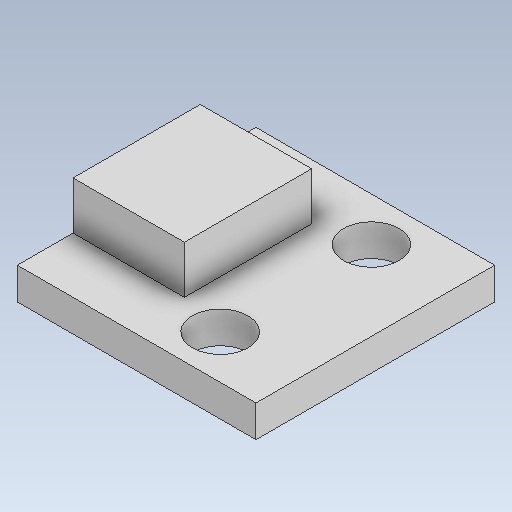
# Autodesk Inventor part: Charger_Port
Saved by Autodesk Inventor 2020 (Build 240168000, 168)
## iProperties
Created: 2021-11-16
Part Number: Charger_Port
Material: Generic
Document SubType Name: Modeling
Designer: mtkts
Density: 1 g/cm^3
Appearance: Default
Author: mtkts
Autodesk Inventor part; units mm, degrees
ref_plane "YZ Plane" through (0, 0, 0) normal (1, 0, 0) x (0, 1, 0)
ref_plane "XZ Plane" through (0, 0, 0) normal (0, 1, 0) x (-1, 0, 0)
ref_plane "XY Plane" through (0, 0, 0) normal (0, 0, 1) x (1, 0, 0)
sketch "Sketch1" plane through (0, 0, 0) normal (0, 1, 0) x (-1, 0, 0)
  line L0 (-7.5, 7.5) -> (7.5, 7.5)
  line L1 (7.5, 7.5) -> (7.5, -7.5)
  line L2 (7.5, -7.5) -> (-7.5, -7.5)
  line L3 (-7.5, -7.5) -> (-7.5, 7.5)
  line L4 (-7.5, 7.5) -> (7.5, -7.5) construction
  line L5 (7.5, 7.5) -> (-7.5, -7.5) construction
  point P0 (0, 0)
  dimension "d0" = 15
  dimension "d1" = 15
  constraints: 12 end point, 2 midpoint, 2 parallel, 1 horizontal, 1 perpendicular
  measures "d0" distance of L1.end L2.end
  measures "d1" distance of L0.end L1.end
extrude "Extrusion1" add sketch "Sketch1" along normal blind 2
sketch "Sketch2" plane through (0, 2, 0) normal (0, 1, 0) x (1, 0, 0)
  line L0 (7.5, 7.5) -> (-7.5, 7.5) construction
  line L1 (-7.5, 7.5) -> (-7.5, -7.5) construction
  line L2 (-7.5, -7.5) -> (7.5, -7.5) construction
  line L3 (7.5, -7.5) -> (7.5, 7.5) construction
  line L4 (-7.5, 7.5) -> (-7.5, -7.5) projected
  line L5 (-7.5, 0) -> (-0.5, 0)
  line L6 (-0.5, 0) -> (-0.5, 4)
  line L7 (-0.5, 4) -> (-7.5, 4)
  line L8 (-7.5, 4) -> (-7.5, 0)
  line L9 (-7.5, 0) -> (-0.5, 0) construction
  line L10 (-7.5, 0) -> (-0.5, 0)
  line L11 (-0.5, 0) -> (-0.5, -4)
  line L12 (-0.5, -4) -> (-7.5, -4)
  line L13 (-7.5, -4) -> (-7.5, 0)
  point P0 (0, 0)
  point P1 (-7.5, 4)
  dimension "d4" = 7
  dimension "d5" = 0
  dimension "d6" = 4
  dimension "d7" = 4
  constraints: 18 end point, 5 equal length, 3 perpendicular, 1 collinear, 1 horizontal, 1 midpoint
  measures "d4" distance of L5.start L5.end
  measures "d5" distance between parallel lines of L5 L9
  measures "d6" distance of L6.end L5.end
  measures "d7" distance of L9.end L11.end
extrude "Extrusion2" add sketch "Sketch2" along normal blind 3
sketch "Sketch3" plane through (0, 2, 0) normal (0, 1, 0) x (1, 0, 0)
  line L0 (-0.5, 4) -> (-0.5, -4) construction
  line L1 (7.5, 7.5) -> (-7.5, 7.5) construction
  line L2 (7.5, 4.75) -> (2.5, 4.75) construction
  circle A0 centre (2.5, 4.75) radius 1.75
  line L3 (7.5, -7.5) -> (7.5, 7.5) construction
  line L4 (0, 0) -> (7.5, 0) construction
  line L5 (7.5, -7.5) -> (7.5, 7.5) construction
  circle A1 centre (2.5, -4.75) radius 1.75
  dimension "d10" = 5
  dimension "d11" = 3.5
  dimension "d12" = 2.75
  constraints: 4 end point, 2 centre point, 1 coincident, 1 midpoint, 1 perpendicular, 1 point on line, 1 symmetric about line, 1 other
  measures "d10" distance of L2.start L2.end
  measures "d11" diameter of A0
  measures "d12" distance from line of L1 L2.end
extrude "Extrusion3" cut sketch "Sketch3" against normal through all
equation "\"d7\" = d6"
body "Solid1"
